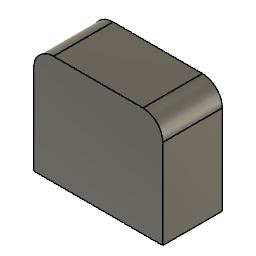
cover_motor_top (Autodesk Fusion 360 design; units mm, degrees)
Autodesk Fusion 360 part; units mm, degrees
sketch "Sketch1" plane through (0, 0, 0) normal (0, 1, 0) x (1, 0, 0)
  line L0 (25.6354, -40) -> (70.6354, -40)
  line L1 (80.6354, -30) -> (80.6354, 15)
  line L2 (80.6354, 15) -> (15.6354, 15)
  line L3 (15.6354, 15) -> (15.6354, -30)
  arc A0 (15.6354, -30) -> (25.6354, -40) centre (25.6354, -30) ccw
  arc A1 (70.6354, -40) -> (80.6354, -30) centre (70.6354, -30) ccw
  dimension "d1" = 65
  dimension "d2" = 55
  dimension "d3" = 10
  dimension "d4" = 10
  constraint horizontal L0
  constraint vertical L1
  constraint horizontal L2
  constraint vertical L3
  constraint tangent L0 A0
  constraint tangent L3 A0
  constraint tangent L0 A1
  constraint tangent L1 A1
  measures "d1" distance of L1 L3
  measures "d2" distance of L0 L2
  measures "d3" radius of A0
  measures "d4" radius of A1
extrude "Extrude2" add sketch "Sketch1" along normal blind 30
shell "Shell2" thickness 3 removed faces 1 at (58.9688, 20, -15)
sketch "Sketch2" plane through (0, 0, 0) normal (1, 0, 0) x (0, 1, 0)
  line L0 (21, 15.6496) -> (10, 15.6496)
  line L1 (10, 15.6496) -> (10, -16.8071)
  line L2 (10, -16.8071) -> (21, -16.8071)
  line L3 (21, -16.8071) -> (21, 15.6496)
  dimension "d11" = 11
  constraint horizontal L0
  constraint vertical L1
  constraint horizontal L2
  constraint vertical L3
  measures "d11" distance of L1 L3
extrude "Extrude3" cut sketch "Sketch2" along normal blind 25
